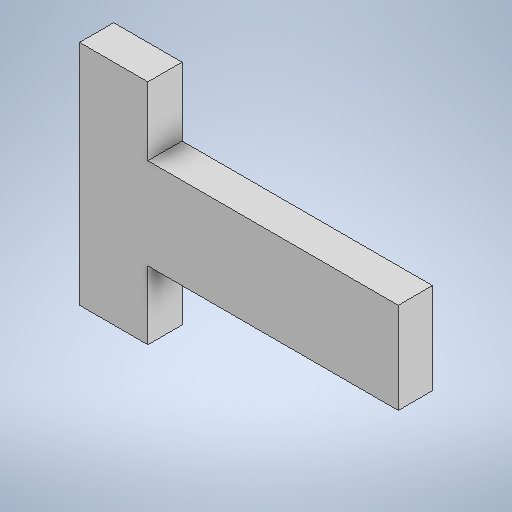
# Autodesk Inventor part: Select Holding Pins
Saved by Autodesk Inventor 2025.3 (Build 293356000, 356)
## iProperties
Created: 2026-04-27
Part Number: Select Holding Pins
Material: Generic
Document SubType Name: Modeling
Designer: kamal
Density: 1 g/cm^3
Appearance: Default
Author: kamal
Autodesk Inventor part; units mm, degrees
ref_plane "YZ Plane" through (0, 0, 0) normal (1, 0, 0) x (0, 1, 0)
ref_plane "XZ Plane" through (0, 0, 0) normal (0, 1, 0) x (-1, 0, 0)
ref_plane "XY Plane" through (0, 0, 0) normal (0, 0, 1) x (1, 0, 0)
sketch "Sketch1" plane through (0, 0, 0) normal (0, 0, 1) x (1, 0, 0)
  line L0 (0, 0) -> (3, 0) construction
  line L1 (25, 0) -> (25, 8)
  line L2 (25, 8) -> (3, 8)
  line L3 (0, 8) -> (0, 0) construction
  line L4 (-3, -6) -> (3, -6)
  line L5 (3, -6) -> (3, 0)
  line L6 (3, 14) -> (-3, 14)
  line L7 (-3, 14) -> (-3, -6)
  line L8 (-3, -6) -> (3, 14) construction
  line L9 (3, -6) -> (-3, 14) construction
  line L10 (3, 8) -> (3, 14)
  line L11 (3, 0) -> (3, 8) construction
  line L12 (3, 8) -> (0, 8) construction
  line L13 (3, 0) -> (25, 0)
  point P0 (0, 4)
  dimension "d0" = 25
  dimension "d1" = 8
  dimension "d2" = 6
  dimension "d3" = 20
  constraints: 28 end point, 9 parallel, 5 perpendicular, 3 horizontal, 3 midpoint
  measures "d0" distance of L3.start L1.end
  measures "d1" distance of L1.end L1.start
  measures "d2" distance of L6.end L6.start
  measures "d3" distance of L6.start L4.end
extrude "Extrusion1" add sketch "Sketch1" along normal blind 3
body "Solid1"
